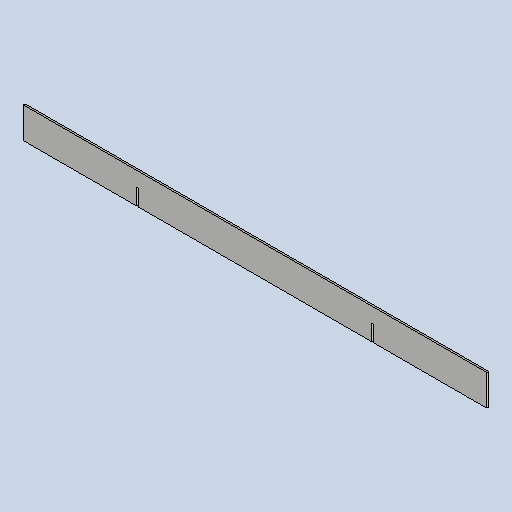
# Autodesk Inventor part: MSC 107 rib cone
Saved by Autodesk Inventor 2025 (Build 290162010, 162A)
## iProperties
Created: 2024-06-26
Part Number: MSC 107 rib cone
Material: Stainless Steel
Document SubType Name: Sheet Metal
Designer: pokla
Density: 8 g/cm^3
Sheet Metal Rule: AISI304 3mm Die 32
Appearance: Default
Stock Number: МОО 107 шпангоут конус
Author: pokla
Autodesk Inventor part; units mm, degrees
ref_plane "YZ Plane" through (0, 0, 0) normal (1, 0, 0) x (0, 1, 0)
ref_plane "XZ Plane" through (0, 0, 0) normal (0, 1, 0) x (-1, 0, 0)
ref_plane "XY Plane" through (0, 0, 0) normal (0, 0, 1) x (1, 0, 0)
sketch "Sketch2" plane through (0, 0, 0) normal (0, 1, 0) x (-1, 0, 0)
  line L0 (375, 50) -> (-375, 50)
  line L1 (-375, 50) -> (-375, 0)
  line L2 (-375, 0) -> (375, 0)
  line L3 (375, 0) -> (375, 50)
  circle A0 centre (-375, 0) radius 22.5
  circle A1 centre (375, 0) radius 22.5
  point P0 (0, 0)
  point P1 (0, 0)
  point P2 (-375, 22.5)
  point P3 (-352.5, 0)
  point P4 (352.5, 0)
  point P5 (375, 22.5)
  dimension "d18" = 750
  dimension "d19" = 50
  dimension "d20" = 45
  measures "d18" distance of L2.end L1.end
  measures "d19" distance of L1.end L0.end
  measures "d20" diameter of A0
extrude "Plate2" add sketch "Sketch2" along normal blind 3 contours L3 A1 L2 A0 L1 L0 | L3 L2 A1 | A0 L2 L1 picked at (360.188, 1.6689) picked at (-360.9308, 4.923)
sketch "Sketch3" plane through (0, 3, 0) normal (0, 1, 0) x (1, 0, 0)
  line L0 (-190, 0) -> (-190, -50) construction
  line L1 (-375, -50) -> (375, -50) projected
  line L2 (-375, -50) -> (-375, 0) projected
  line L3 (-191.5, 0) -> (-188.5, 0)
  line L4 (-188.5, 0) -> (-188.5, -26)
  line L5 (-188.5, -26) -> (-191.5, -26)
  line L6 (-191.5, -26) -> (-191.5, 0)
  line L7 (-375, 0) -> (375, 0) projected
  line L8 (375, 0) -> (-375, 0) projected
  line L9 (190, 0) -> (190, -50) construction
  line L10 (191.5, -26) -> (188.5, -26)
  line L11 (188.5, -26) -> (188.5, 0)
  line L12 (188.5, 0) -> (191.5, 0)
  line L13 (191.5, 0) -> (191.5, -26)
  point P0 (0, 0)
  point P1 (-330, -22.5)
  point P2 (-307.5, 0)
  point P3 (307.5, 0)
  point P4 (0, 0)
  point P5 (0, 0)
  point P6 (188.5, 0)
  dimension "d23" = 3
  dimension "d24" = 26
  dimension "d30" = 190
  dimension "d31" = 190
  dimension "d32" = 3
  dimension "d33" = 26
  constraints: 20 end point, 4 parallel, 3 midpoint, 3 perpendicular, 3 point on line, 2 horizontal, 1 vertical, 4 other
  measures "d23" distance of L3.start L3.end
  measures "d24" distance of L3.end L4.end
  measures "d30" distance from line of point (0, 0) L0
  measures "d31" distance from line of point (0, 0) L9
  measures "d32" distance of L11.end L12.end
  measures "d33" distance of L12.end L10.start
extrude "Extrusion1" cut sketch "Sketch3" against normal through all
equation "\"d23\" = Thickness"
equation "\"d31\" = d30"
equation "\"d32\" = Thickness"
equation "\"d33\" = d24"
equation "\"d21\" = Thickness"
equation "\"BendReliefWidth\" = Thickness"
equation "\"BendReliefDepth\" = 0.5 * Thickness"
equation "\"CornerReliefSize\" = 4 * Thickness"
equation "\"MinimumRemnant\" = 2 * Thickness"
equation "\"TransitionRadius\" = BendRadius"
equation "\"JacobiRadiusSize\" = BendRadius"
equation "\"GapSize\" = Thickness"
equation "\"Thickness\" = 3"
equation "\"BendRadius\" = 5"
body "Solid2"
